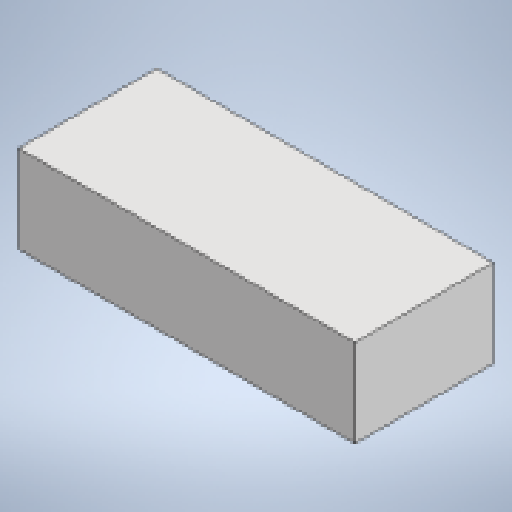
# Autodesk Inventor part: Temp - Battery
Saved by Autodesk Inventor 2023.2 (Build 272271000, 271)
## iProperties
Created: 2023-06-09
Part Number: Temp - Battery
Material: Generic
Document SubType Name: Modeling
Designer: Nathan Cai
Mass: 70.5 g
Surface Area: 82.94 cm^2
Volume: 41.61 cm^3
Density: 1.6943 g/cm^3
Appearance: Default
Author: Nathan Cai
Autodesk Inventor part; units mm, degrees
ref_plane "YZ Plane" through (0, 0, 0) normal (1, 0, 0) x (0, 1, 0)
ref_plane "XZ Plane" through (0, 0, 0) normal (0, 1, 0) x (-1, 0, 0)
ref_plane "XY Plane" through (0, 0, 0) normal (0, 0, 1) x (1, 0, 0)
sketch "Sketch1" plane through (0, 0, 0) normal (0, 1, 0) x (-1, 0, 0)
  line L0 (0, 0) -> (73, 0)
  line L1 (73, 0) -> (73, -30)
  line L2 (73, -30) -> (0, -30)
  line L3 (0, -30) -> (0, 0)
  dimension "d0" = 73
  dimension "d1" = 30
  constraints: 8 end point, 2 parallel, 1 horizontal, 1 perpendicular
  measures "d0" distance of L1.end L2.end
  measures "d1" distance between parallel lines of L0 L2
extrude "Extrusion1" add sketch "Sketch1" along normal blind 19
body "Solid1"
